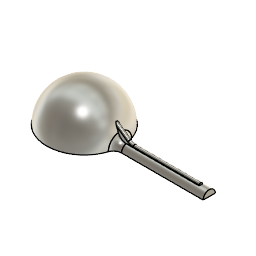
EchoWeather_WindCup v3 (Autodesk Fusion 360 design; units mm, degrees)
Autodesk Fusion 360 part; units mm, degrees
note: some values were not read from the file. Chosen so that the rebuilt part matches the saved one: which face or edge a step refers to.
sketch "Sketch2" plane through (0, 0, 0) normal (0, 1, 0) x (1, 0, 0)
  line L0 (0, 0) -> (0, -28.575) construction
  line L1 (0, 0) -> (29.575, 0) construction
  line L2 (29.575, 0) -> (28.575, 0)
  line L3 (0, -28.575) -> (0, -29.575)
  arc A0 (0, -28.575) -> (28.575, 0) centre (0, 0) ccw
  arc A1 (0, -29.575) -> (29.575, 0) centre (0, 0) ccw
  dimension "d1" = 28.575
  dimension "d3" = 29.575
  constraint coincident L0.start L1.start
  constraint vertical L0
  constraint perpendicular L0 L1
  constraint coincident L1 L2.end
  constraint perpendicular L2 L3
  measures "d1" distance of L0.start L0.end
  measures "d3" distance of L0.start L1.end
revolve "Revolve1" add sketch "Sketch2" angle 360 about axis through (0, 0, 0) along (0, 0, 1)
sketch "Sketch3" plane through (0, 0, 0) normal (1, 0, 0) x (0, 1, 0)
  line L0 (4.826, 0) -> (-4.826, 0)
  arc A0 (4.826, 0) -> (-4.826, 0) centre (0, 0) ccw
  line L1 (0, 0) -> (-9.077252, 0) construction
  dimension "d5" = 9.652
  constraint coincident A0.centre L1.start
  constraint horizontal L0
  constraint horizontal L1
  constraint collinear L0 L1
  measures "d5" diameter of A0
extrude "Extrude1" add sketch "Sketch3" along normal blind 69.85 from surface at 28.575
fillet "Fillet1" radius 6.35 2 edges at (29.178594, 3.41241, 3.412585) (29.178594, -3.412497, 3.412498)
sketch "Sketch5" plane through (0, 0, 0) normal (0, 1, 0) x (1, 0, 0)
  line L0 (34.142388, 0) -> (34.142388, -4.826) construction
  line L1 (34.142388, 0) -> (98.425, 0) construction
  line L2 (98.425, -4.826) -> (98.425, 0) construction
  line L3 (98.425, 0) -> (34.142388, 0) construction
  line L4 (34.142388, 0) -> (28.107477, 0) construction
  line L5 (34.142388, 0) -> (34.142388, -4.826) construction
  line L6 (34.142388, 0) -> (28.107477, 0) construction
  line L7 (28.107477, -9.200562) -> (28.107477, 0) construction
  line L8 (28.107477, -9.200562) -> (28.107477, 0) construction
  line L9 (-29.575, 0) -> (28.107477, 0) construction
  line L10 (98.425, -4.826) -> (91.821, -4.826) construction
  line L11 (91.821, -4.826) -> (34.142388, -4.826)
  line L12 (91.821, -4.826) -> (91.821, -6.4135)
  line L13 (91.821, -6.4135) -> (39.848147, -6.4135)
  line L14 (36.205937, -7.561885) -> (25.422116, -15.112797)
  arc A0 (25.422116, -15.112797) -> (28.107477, -9.200562) centre (0, 0) ccw
  arc A1 (39.848147, -6.4135) -> (36.205937, -7.561885) centre (39.848147, -12.7635) ccw
  arc A2 (34.142388, -4.826) -> (28.107477, -9.200562) centre (34.142388, -11.176001) ccw
  line L15 (91.821, -4.064) -> (34.142389, -4.064)
  arc A3 (34.142389, -4.064) -> (27.383288, -8.96351) centre (34.142388, -11.176001) ccw
  arc A4 (24.767661, -14.722498) -> (27.383288, -8.96351) centre (0, 0) ccw
  line L16 (24.767661, -14.722498) -> (25.422116, -15.112797)
  line L17 (91.821, -4.826) -> (91.821, -4.064)
  point P0 (37.846, -6.4135)
  dimension "d18" = 6.604
  dimension "d19" = 1.5875
  dimension "d20" = 145
  dimension "d21" = 53.975
  dimension "d22" = 6.35
  dimension "d23" = -0.762
  constraint coincident A0.centre A4.centre
  constraint coincident L2.start L10.start
  constraint perpendicular L2 L10
  constraint perpendicular L10 L12
  constraint perpendicular L12 L13
  constraint coincident P0 L14
  constraint coincident P0 L13
  constraint tangent L14 A1
  constraint tangent L13 A1
  constraint tangent A0 A2
  constraint perpendicular L10 L17
  measures "d18" distance of L2.start L10.end
  measures "d19" distance of L10.end L12.end
  measures "d20" angle of L13 L14
  measures "d21" distance of L12.end P0
  measures "d22" radius of A1
extrude "Extrude3" add sketch "Sketch5" along normal blind 2.54 from surface at -1.27
fillet "Fillet2" radius 1.27 6 edges at (65.834574, -1.27, 6.4135) (37.938665, -1.27, 6.707397) (30.814027, -1.27, 11.337341) (30.814027, 1.27, 11.337341) (37.938665, 1.27, 6.707397) (65.834574, 1.27, 6.4135)
equation "d3 = 1.125 in + 1 mm"
